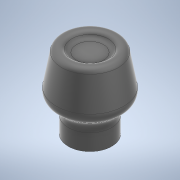
# Autodesk Inventor part: 08-02-01-011_funkyKnob
Saved by Autodesk Inventor 2020 (Build 240168000, 168)
## iProperties
Created: 2021-08-25
Part Number: 08-02-01-011_funkyKnob
Material: ABS-Kunststoff(1)
Document SubType Name: Modeling
Designer: Eric
Density: 1.06 g/cm^3
Appearance: Glatt - Weiß(1)
Author: Eric
## iProperties of the stored document _3D-Druck.ipt
Created: 2021-08-28
Part Number: _3D-Druck
Material: Generisch
Document SubType Name: Modeling
Designer: Eric
Density: 1 g/cm^3
Appearance: Vorgabe
Author: Eric
Autodesk Inventor part; units mm, degrees
ref_plane "YZ Plane" through (0, 0, 0) normal (1, 0, 0) x (0, 1, 0)
ref_plane "XZ Plane" through (0, 0, 0) normal (0, 1, 0) x (-1, 0, 0)
ref_plane "XY Plane" through (0, 0, 0) normal (0, 0, 1) x (1, 0, 0)
sketch "Skizze2" plane through (0, 0, 0) normal (1, 0, 0) x (0, 1, 0)
  line L0 (13, 0) -> (0, 0)
  line L1 (3, 4) -> (0, 4)
  line L2 (0, 4) -> (0, 0)
  line L3 (5.9544, 6.4791) -> (13.1736, 5.2061)
  line L4 (13.1736, 5.2061) -> (5.9544, 6.4791)
  arc A0 (3, 4) -> (5.9544, 6.4791) centre (3, 7) ccw
  arc A1 (13.5, 3.3553) -> (13.1736, 5.2061) centre (13, 4.2213) ccw
  arc A2 (13.5, 3.3553) -> (13, 2.4893) centre (14, 2.4893) ccw
  line L5 (13, 2.4893) -> (13, 0)
  dimension "d3" = 80
  dimension "d4" = 4
  dimension "d5" = 13
  dimension "d7" = 3
  dimension "d8" = 1
  dimension "d9" = 3
  dimension "d10" = 0
  constraints: 13 end point, 6 point on circle, 4 tangent, 3 centre point, 2 perpendicular, 1 coincident, 1 equal radius, 1 horizontal, 1 line through centre, 1 vertical
  measures "d3" angle of L2 L3
  measures "d4" distance of L1.end L0.end
  measures "d5" distance of L0.start L0.end
  measures "d7" radius of A0
  measures "d8" radius of A1
  measures "d9" distance of L1.start L1.end
  measures "d10" distance from line of L5 A1.centre
revolve "Umdrehung1" add sketch "Skizze2" angle 360 about axis through (0, 13, 0) along (0, -1, 0)
sketch "Skizze1" plane through (0, 0, 0) normal (0, 1, 0) x (-1, 0, 0)
  arc A0 (-1.1779, 0.55) -> (1.1779, 0.55) centre (0, 0) ccw
  line L0 (-1.1779, 0.55) -> (1.1779, 0.55)
  dimension "d0" = 1.3
  dimension "d1" = 0.55
  constraints: 3 point on circle, 2 end point, 1 centre point, 1 coincident, 1 horizontal, 1 horizontal alignment
  measures "d0" radius of A0
  measures "d1" distance from line of point (0, 0) L0
extrude "Extrusion1" cut sketch "Skizze1" along normal blind 6
sketch "Skizze3" plane through (0, 0, 0) normal (0, -1, 0) x (1, 0, 0)
  arc A0 (-1.1779, 0.55) -> (1.1779, 0.55) centre (0, 0) ccw projected
  circle A1 centre (0, 0) radius 1.5
  point P0 (0, 0)
  dimension "d14" = 3
  constraints: 1 centre point, 1 coincident
  measures "d14" diameter of A1
extrude "Extrusion2" cut sketch "Skizze3" against normal blind 1
fillet "Rundung1" radius 2 1 edges at (0, 5.9544, -6.4791)
